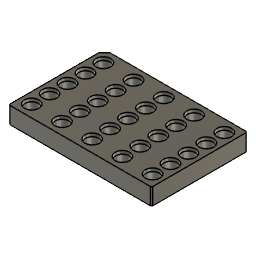
vialtrayholder_25_tuberack_1000ul (Autodesk Fusion 360 design; units mm, degrees)
Autodesk Fusion 360 part; units mm, degrees
sketch "Sketch1" plane through (0, 0, 0) normal (0, 0, 1) x (1, 0, 0)
  line L0 (63.85, 42.75) -> (-63.85, 42.75)
  line L1 (-63.85, 42.75) -> (-63.85, -42.75)
  line L2 (-63.85, -42.75) -> (63.85, -42.75)
  line L3 (63.85, -42.75) -> (63.85, 42.75)
  line L4 (63.85, 42.75) -> (-63.85, -42.75) construction
  line L5 (-63.85, 42.75) -> (63.85, -42.75) construction
  dimension "d1" = 127.7
  dimension "d2" = 85.5
  constraint horizontal L0
  constraint perpendicular L0 L1
  constraint parallel L0 L2
  constraint parallel L1 L3
  constraint coincident L4 origin
  constraint coincident L5 origin
  measures "d1" distance of L1.end L2.end
  measures "d2" distance of L0.end L1.end
extrude "Extrude1" add sketch "Sketch1" along normal blind 15
sketch "Sketch6" plane through (0, 0, 15) normal (0, 0, 1) x (-1, 0, 0)
  line L0 (-63.85, 42.75) -> (-63.85, -42.75)
  line L1 (-63.85, -42.75) -> (63.85, -42.75)
  line L2 (63.85, -42.75) -> (63.85, 42.75)
  line L3 (63.85, 42.75) -> (-63.85, 42.75)
  point P0 (54, -32)
  point P1 (27, -32)
  point P2 (0, -32)
  point P3 (-27, -32)
  point P4 (54, -16)
  point P5 (27, -16)
  point P6 (0, -16)
  point P7 (-27, -16)
  point P8 (54, 0)
  point P9 (27, 0)
  point P10 (-27, 0)
  point P11 (54, 16)
  point P12 (27, 16)
  point P13 (0, 16)
  point P14 (-27, 16)
  point P15 (54, 32)
  point P16 (27, 32)
  point P17 (0, 32)
  point P18 (-27, 32)
  point P19 (-54, -32)
  point P20 (-54, -16)
  point P21 (-54, 0)
  point P22 (-54, 16)
  point P23 (-54, 32)
  dimension "d37" = 16
hole "Hole2" at (-54, 32, 15) direction (0, 0, -1) diameter 12.05 depth 12.5 tip angle 180
chamfer "Chamfer4" distance 0.5 distance2 2.5 1 edges at (-59.6173, 34.1787, 15) measured on face at (26.3059, 9.6625, 15)
pattern_linear "R-Pattern1" count 5 spacing 27 along (1, 0, 0) count 5 spacing 16 along (0, -1, 0) of "Hole2", "Chamfer4"
chamfer "Chamfer3" distance 5 angle 45 1 edges at (-63.85, 42.75, 7.5)
chamfer "Chamfer3" distance 1 angle 45 3 edges at (-63.85, -42.75, 7.5) (63.85, -42.75, 7.5) (63.85, 42.75, 7.5)
equation "num_x = 5"
equation "num_y = 5"
equation "hole_spacing_x = 27 mm"
equation "vial_diameter = 11.8 mm"
equation "d30 = vial_diameter + 0.25 mm"
equation "d34 = num_x"
equation "d35 = num_y"
equation "d36 = -hole_spacing_x"
equation "d37 = hole_spacing_y"
equation "d38 = num_x"
equation "d39 = num_y"
equation "d40 = hole_spacing_x"
equation "d41 = hole_spacing_y"
equation "hole_spacing_y = 16 mm"
